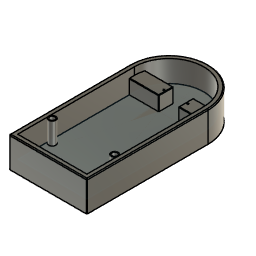
Baseplate(x1) (Autodesk Fusion 360 design; units mm, degrees)
Autodesk Fusion 360 part; units mm, degrees
note: some values were not read from the file. Set by a fixed rule: which sketch regions a step uses.
sketch "Sketch1" plane through (0, 0, 0) normal (0, 0, 1) x (1, 0, 0)
  line L0 (-45, 0) -> (45, 0)
  line L1 (45, 0) -> (45, -140)
  line L2 (45, -140) -> (-45, -140)
  line L3 (-45, -140) -> (-45, 0)
  line L4 (-40, 0) -> (40, 0)
  line L5 (40, 0) -> (40, -135)
  line L6 (40, -135) -> (-40, -135)
  line L7 (-40, -135) -> (-40, 0)
  arc A0 (45, 0) -> (-45, 0) centre (0, 0) ccw
  arc A1 (40, 0) -> (-40, 0) centre (0, 0) ccw
  dimension "d1" = 90
  dimension "d2" = 80
  dimension "d3" = 140
  dimension "d4" = 135
  constraint coincident A0.centre A1.centre
  constraint perpendicular L0 L1
  constraint parallel L0 L2
  constraint parallel L1 L3
  constraint horizontal L0
  constraint tangent L3 A0
  constraint perpendicular L4 L5
  constraint parallel L4 L6
  constraint parallel L5 L7
  constraint coincident L0 L4.end
  constraint parallel L0 L4
  measures "d1" diameter of A0
  measures "d2" diameter of A1
  measures "d3" distance of L0.start L2.end
  measures "d4" distance of L4.start L6.end
extrude "Extrude1" add sketch "Sketch1" along normal blind 35.1 contours L0 A0 A1 | L0 L1 L2 L3 L5 L6 L7 makes body 1
extrude "Extrude2" add sketch "Sketch1" along normal blind 10 separate body contours L0 L4 A1 | L0 L4 L5 L6 L7 makes body 2
sketch "Sketch2" plane through (0, 0, 10) normal (0, 0, 1) x (-1, 0, 0)
  line L0 (-40, 135) -> (-40, 0)
  arc A0 (-40, 0) -> (40, 0) centre (0, 0) ccw
  line L1 (40, 0) -> (40, 135)
  line L2 (40, 135) -> (-40, 135)
sketch "Sketch3" plane through (0, 0, 10) normal (0, 0, 1) x (-1, 0, 0)
  line L0 (40, 0) -> (40, 6)
  arc A0 (-40, 0) -> (40, 0) centre (0, 0) ccw
  line L1 (24, -11) -> (6, -11)
  line L2 (6, -11) -> (6, 6)
  line L3 (6, 6) -> (40, 6)
  line L4 (0, 0) -> (0, -20)
  line L5 (0, -20) -> (0, 17)
  line L6 (0, 0) -> (0, -20)
  line L7 (0, -20) -> (0, 17)
  line L8 (-16.8, 6) -> (-40, 6)
  line L9 (-40, 0) -> (-40, 6)
  line L10 (-24.0196, -11) -> (-16.8, -11)
  line L11 (-16.8, -11) -> (-16.8, 6)
  line L12 (0, 0) -> (40, 0) construction
  line L13 (0, 0) -> (-40, 0) construction
  line L14 (24, -11) -> (38.4578, -11)
  line L15 (-24.0196, -11) -> (-38.4578, -11)
  dimension "d9" = 6
  dimension "d22" = 34
  dimension "d23" = 23.2
  dimension "d30" = 11
  dimension "d32" = 17
  dimension "d49" = 22.8
  constraint vertical L0
  constraint perpendicular L1 L2
  constraint coincident A0.centre L4.start
  constraint vertical L4
  constraint parallel L4 L5
  constraint symmetric L0.start L5 A0.start
  constraint symmetric L0.end L5 L8.end
  constraint symmetric A0.centre L5 L4.start
  constraint symmetric L4.end L5 L6.end
  constraint symmetric L7.end L5 L5.end
  constraint perpendicular L0 L3
  constraint perpendicular L2 L3
  constraint perpendicular L8 L11
  constraint perpendicular L10 L11
  constraint coincident L0.start A0.end
  constraint perpendicular L9 L13
  constraint coincident A0 L14.end
  constraint coincident A0 L15.end
  constraint parallel L1 L14
  constraint parallel L10 L15
  constraint parallel L2 L11
  measures "d9" distance of L0.start L0.end
  measures "d22" distance of L0.end L2.end
  measures "d23" distance of L8.start L8.end
  measures "d30" distance of L1 L12
  measures "d32" distance of L8 L10
  measures "d49" distance of L2 L11
extrude "Extrude3" add sketch "Sketch3" along normal blind 16.5 bodies 1 2
sketch "Sketch4" plane through (0, 0, 26.5) normal (0, 0, 1) x (-1, 0, 0)
  line L0 (40, 0) -> (40, 6)
  line L1 (40, 6) -> (6, 6)
  line L2 (6, 6) -> (6, -11)
  line L3 (6, -11) -> (38.4578, -11)
  line L4 (6, -11) -> (6, -2.5)
  line L5 (6, -2.5) -> (10.7, -2.5)
  line L6 (10.7, -2.5) -> (8.4, -2.5)
  circle A0 centre (8.4, -2.5) radius 1.05
  line L7 (-16.8, -11) -> (-16.8, -2.5)
  line L8 (-16.8, -2.5) -> (-21.5, -2.5)
  line L9 (-21.5, -2.5) -> (-19.2, -2.5)
  circle A1 centre (-19.2, -2.5) radius 1.05
  line L10 (-38.4578, -11) -> (-16.8, -11)
  line L11 (-16.8, -11) -> (-16.8, 6)
  arc A2 (38.4578, -11) -> (40, 0) centre (0, 0) ccw
  dimension "d14" = 8.5
  dimension "d15" = 4.7
  dimension "d16" = 2.3
  dimension "d17" = 2.1
  dimension "d24" = 8.5
  dimension "d25" = 4.7
  dimension "d26" = 2.3
  dimension "d27" = 2.1
  constraint coincident L2.end L3.start
  constraint perpendicular L1 L4
  constraint perpendicular L4 L5
  constraint perpendicular L2 L6
  constraint coincident L6.end A0.centre
  constraint vertical L7
  constraint perpendicular L7 L8
  constraint parallel L8 L9
  constraint coincident L9.end A1.centre
  constraint coincident L7.start L10
  constraint coincident L7.start L11
  measures "d14" distance of L2.end L4.end
  measures "d15" distance of L4.end L5.end
  measures "d16" distance of L5.end L6.end
  measures "d17" diameter of A0
  measures "d24" distance of L7.start L7.end
  measures "d25" distance of L7.end L8.end
  measures "d26" distance of L8.end L9.end
  measures "d27" diameter of A1
extrude "Extrude4" cut sketch "Sketch4" against normal blind 8 contours L5 L6 A0 | L5 L6 A0 bodies 1
extrude "Extrude5" cut sketch "Sketch4" against normal blind 8 contours L8 L9 A1 | L8 L9 A1 bodies 1
fillet "Fillet1" radius 0.5 1 edges at (16.8, 2.5, 26.5) on bodies 1
fillet "Fillet2" radius 0.5 3 edges at (27.8789, 11, 26.5) (16.9464, 11, 26.3536) (16.8, 11, 18) on bodies 1
fillet "Fillet3" radius 0.5 3 edges at (16.8, -6, 18) (16.9464, -6, 26.3536) (28.65, -6, 26.5) on bodies 1
fillet "Fillet4" radius 0.5 1 edges at (-23, -6, 26.5) on bodies 1
fillet "Fillet5" radius 0.5 3 edges at (-6, -6, 18) (-6, -5.8536, 26.3536) (-6, 2.75, 26.5) on bodies 1
fillet "Fillet6" radius 0.5 3 edges at (-6, 11, 18) (-6.1464, 11, 26.3536) (-22.4789, 11, 26.5) on bodies 1
fillet "Fillet7" radius 1 5 edges at (-45, -140, 17.55) (0, -140, 35.1) (45, -70, 35.1) (0, 45, 35.1) (-45, -70, 35.1) on bodies 1
fillet "Fillet8" radius 0.5 2 edges at (45, -140, 17.05) (44.7071, -139.7071, 34.8071) on bodies 1
sketch "Sketch5" plane through (0, 0, 10) normal (0, 0, 1) x (-1, 0, 0)
  line L0 (40, 135) -> (40, 95)
  circle A0 centre (36, 99) radius 4
  circle A1 centre (-36, 99) radius 4
  line L1 (-40, 135) -> (-40, 95)
  line L2 (40, 135) -> (-40, 135)
  point P0 (40, 135)
  point P1 (-40, 135)
  dimension "d50" = 40
  dimension "d51" = 8
  dimension "d52" = 8
  dimension "d53" = 40
  dimension "d54" = 36
  dimension "d55" = 36
  constraint vertical L0
  constraint tangent L0 A0
  constraint vertical L1
  constraint tangent A1 L1
  constraint coincident P0 L0.start
  constraint coincident P1 L1.start
  measures "d50" distance of P0 L0.end
  measures "d51" diameter of A0
  measures "d52" diameter of A1
  measures "d53" distance of P1 L1.end
  measures "d54" distance of A0.centre L2
  measures "d55" distance of A1.centre L2
extrude "Extrude6" add sketch "Sketch5" along normal blind 25 thin wall 1 inside separate body makes body 3 at (32.0199, -98.6017, 18.3333) makes body 4 at (-39.9801, -98.6017, 18.3333)
equation "d5 = 30 mm + 5.1 mm"
